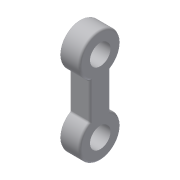
# Autodesk Inventor part: Part2
Saved by Autodesk Inventor 2014 (Build 180170000, 170)
## iProperties
Created: 2013-07-16
Part Number: Part2
Material: Generic
Document SubType Name: Modeling
Density: 1 g/cm^3
Appearance: Default
Autodesk Inventor part; units mm, degrees
ref_plane "YZ Plane" through (0, 0, 0) normal (1, 0, 0) x (0, 1, 0)
ref_plane "XZ Plane" through (0, 0, 0) normal (0, 1, 0) x (-1, 0, 0)
ref_plane "XY Plane" through (0, 0, 0) normal (0, 0, 1) x (1, 0, 0)
sketch "Sketch1" plane through (0, 0, 0) normal (1, 0, 0) x (0, 1, 0)
  circle A0 centre (0, 35) radius 10
  circle A1 centre (0, -35) radius 10
  arc A2 (10, 17.6795) -> (-10, 17.6795) centre (0, 35) ccw
  arc A3 (-10, -17.6795) -> (10, -17.6795) centre (0, -35) ccw
  line L0 (-28.2124, 0) -> (57.6581, 0) construction
  line L1 (-10, 17.6795) -> (-10, -17.6795)
  line L2 (10, 17.6795) -> (10, -17.6795)
  line L3 (0, 0) -> (0, 21.0964) construction
  dimension "d0" = 70
  dimension "d1" = 20
  dimension "d2" = 40
  dimension "d3" = 20
  constraints: 8 end point, 4 centre point, 4 point on circle, 2 coincident, 2 equal radius, 2 horizontal, 2 parallel, 1 perpendicular, 2 other
  measures "d0" distance of A1.centre A0.centre
  measures "d1" diameter of A1
  measures "d2" diameter of A2
  measures "d3" distance between parallel lines of L2 L1
extrude "Extrusion1" add sketch "Sketch1" along normal blind 20
fillet "Fillet1" radius 2 8 edges at (20, 0, 55) (20, 10, 0) (20, -10, 0) (20, 0, -55) (0, 0, -55) (0, 10, 0) (0, 0, 55) (0, -10, 0)
fillet "Fillet2" radius 2 12 edges at (10, 10, 17.6795) (19.4835, 9.3413, 18.0641) (0.5165, 9.3413, 18.0641) (19.4836, 9.3413, -18.0641) (0.5165, 9.3413, -18.0641) (10, 10, -17.6795) (19.4836, -9.3413, 18.0641) (0.5165, -9.3413, 18.0641) (10, -10, 17.6795) (19.4835, -9.3413, -18.0641) (0.5165, -9.3413, -18.0641) (10, -10, -17.6795)
body "Solid1"
